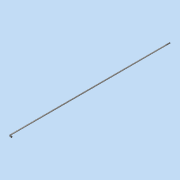
# Autodesk Inventor part: radio
Saved by Autodesk Inventor 2017 (Build 210142000, 142)
## iProperties
Part Number: radio
Material: Acero inoxidable
Document SubType Name: Modeling
Designer: Miguel A.
Density: 8 g/cm^3
Appearance: Semipulido
Author: Miguel A.
Autodesk Inventor part; units mm, degrees
ref_plane "YZ Plane" through (0, 0, 0) normal (1, 0, 0) x (0, 1, 0)
ref_plane "XY Plane" through (0, 0, 0) normal (0, 0, 1) x (1, 0, 0)
sketch "Boceto1" plane through (0, 0, 0) normal (0, 0, 1) x (1, 0, 0)
  line L0 (0, 0) -> (-3, 0)
  arc A0 (-5, 2) -> (-3, 0) centre (-3, 2) ccw
  line L1 (-5, 2) -> (-5, 393)
  dimension "d0" = 391
  dimension "d1" = 2
  dimension "d2" = 5
  constraints: 4 end point, 2 point on circle, 2 tangent, 1 centre point, 1 horizontal, 1 vertical
  measures "d0" distance of L1.start L1.end
  measures "d1" radius of A0
  measures "d2" distance from line of L1 L0.start
ref_plane "Plano de trabajo1" through (-5, 393, 0) normal (0, 1, 0) x (-1, 0, 0)
sketch "Boceto2" plane through (-5, 393, 0) normal (0, 1, 0) x (-1, 0, 0)
  circle A0 centre (0, 0) radius 1.25
  point P0 (-5, 0)
  point P1 (0, 0)
  point P2 (0, 0)
  point P3 (0, 0)
  dimension "d3" = 2.5
  constraints: 1 centre point, 1 coincident
  measures "d3" diameter of A0
sweep "Barrido1" add profiles "Boceto2" path "Boceto1"
sketch "Boceto4" plane through (0, 0, 0) normal (1, 0, 0) x (0, 0, -1)
  point P0 (0, 0)
  point P1 (0, 0)
  constraints: 1 coincident
sketch "Boceto3" plane through (0, 0, 0) normal (1, 0, 0) x (0, 0, -1)
  circle A0 centre (0, 0) radius 2
  point P0 (0, 0)
  dimension "d6" = 4
  constraints: 1 centre point, 1 coincident
  measures "d6" diameter of A0
extrude "Extrusión1" add sketch "Boceto3" along normal blind 0.5
fillet "Empalme1" radius 0.25 1 edges at (0, 1.25, 0)
fillet "Empalme2" radius 0.25 2 edges at (0, 0, 2) (0.5, 0, 2)
thread "Rosca1"
